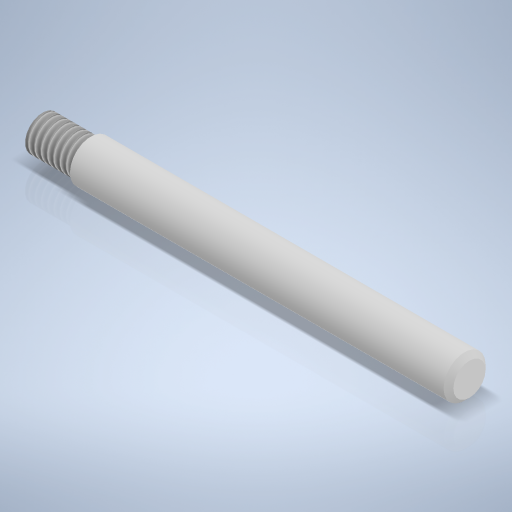
# Autodesk Inventor part: kurbelwelle
Saved by Autodesk Inventor 2024 (Build 280153000, 153)
## iProperties
Created: 2024-04-02
Part Number: kurbelwelle
Material: Generisch
Document SubType Name: Modeling
Designer: ffogue
Density: 1 g/cm^3
Appearance: Vorgabe
Author: ffogue
Autodesk Inventor part; units mm, degrees
ref_plane "YZ Plane" through (0, 0, 0) normal (1, 0, 0) x (0, 1, 0)
ref_plane "XZ Plane" through (0, 0, 0) normal (0, 1, 0) x (-1, 0, 0)
ref_plane "XY Plane" through (0, 0, 0) normal (0, 0, 1) x (1, 0, 0)
sketch "Skizze4" plane through (0, 0, 0) normal (0, 0, 1) x (1, 0, 0)
  line L0 (0, 0) -> (0, 1.25)
  line L1 (0, 1.25) -> (3.4541, 1.25)
  line L2 (3.4541, 1.25) -> (3.4541, 1.5)
  line L3 (3.4541, 1.5) -> (30.5, 1.5)
  line L4 (30.5, 1.5) -> (30.5, 0)
  line L5 (0, 0) -> (30.5, 0)
  dimension "d11" = 30.5
  dimension "d12" = 3
  dimension "d13" = 2.5
  constraints: 12 end point, 4 perpendicular, 1 horizontal, 1 vertical
  measures "d11" distance of L0.start L4.end
  measures "d12" diameter of L3 L5
  measures "d13" diameter of L1 L5
revolve "Umdrehung2" add sketch "Skizze4" angle 360 about axis through (0, 0, 0) along (1, 0, 0)
thread "Gewinde2" size "M2.5x0.45" class "6g" standard "ISO Metric profile" length 4
chamfer "Fasen1" distance 0.35 angle 45 1 edges at (30.5, -1.5, 0)
